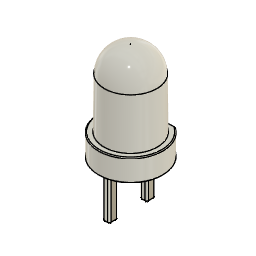
3mm (Autodesk Fusion 360 design; units mm, degrees)
Autodesk Fusion 360 part; units mm, degrees
sketch "Sketch1" plane through (0, 0, 0) normal (0, 0, 1) x (1, 0, 0)
  circle A0 centre (0, 0) radius 1.8
  line L0 (0, 0) -> (0, -1.8)
  line L1 (0, -1.8) -> (0, 1.5)
  line L2 (0, 1.5) -> (-0.995, 1.5)
  line L3 (0, 1.5) -> (0.995, 1.5)
  circle A1 centre (0, 0) radius 1.5
  dimension "d1" = 3.6
  dimension "d2" = 3.3
  dimension "d3" = 3
  constraint coincident A0.centre L0.start
  constraint coincident A0 L0.end
  constraint vertical L0
  constraint parallel L0 L1
  constraint coincident A0 L2.end
  constraint perpendicular L1 L2
  constraint coincident A0 L3.end
  constraint perpendicular L1 L3
  constraint concentric A0 A1
  measures "d1" diameter of A0
  measures "d2" distance of L0.end L1.end
  measures "d3" diameter of A1
extrude "Extrude1" add sketch "Sketch1" along normal blind 5.5 contours L0 L1 A1 | L0 L1 A1
extrude "Extrude2" add sketch "Sketch1" along normal blind 1.25 contours A0 L0 L1 L3 A1 | A0 L0 L1 L2 A1
chamfer "Chamfer1" distance 0.05 distance2 4.25 1 edges at (-1.3985, -0.5424, 5.5) measured on face at (0.4379, -0.6128, 5.5)
fillet "Fillet1" radius 0.05 5 edges at (0, -1.8, 1.25) (0.4975, 1.5, 1.25) (-0.4975, 1.5, 1.25) (0, -1.8, 0) (0, 1.5, 0)
fillet "Fillet2" radius 1.45 1 edges at (-1.3519, 0.5243, 5.5)
sketch "Sketch2" plane through (0, 0, 0) normal (0, 0, -1) x (1, 0, 0)
  line L0 (-0.9798, -1.45) -> (0.9798, -1.45)
  arc A0 (0.9798, -1.45) -> (-0.9798, -1.45) centre (0, 0) ccw
  line L1 (-0.2, -1.2) -> (0.2, -1.2)
  line L2 (0.2, -1.2) -> (0.2, -0.7)
  line L3 (0.2, -0.7) -> (-0.2, -0.7)
  line L4 (-0.2, -0.7) -> (-0.2, -1.2)
  line L5 (-0.2, -1.2) -> (0.2, -0.7) construction
  line L6 (0.2, -1.2) -> (-0.2, -0.7) construction
  line L7 (0, 0) -> (0, -1.45)
  line L8 (0, 0) -> (0, 1.75)
  line L9 (20, 0) -> (2.5, 0)
  arc A1 (0.9487, -1.35) -> (-0.9487, -1.35) centre (0, 0) ccw
  line L10 (-0.9487, -1.35) -> (0.9487, -1.35)
  line L11 (-0.2, 0.9) -> (0.2, 0.9)
  line L12 (0.2, 0.9) -> (0.2, 1.4)
  line L13 (0.2, 1.4) -> (-0.2, 1.4)
  line L14 (-0.2, 1.4) -> (-0.2, 0.9)
  line L15 (-0.2, 0.9) -> (0.2, 1.4) construction
  line L16 (0.2, 0.9) -> (-0.2, 1.4) construction
  point P0 (0, -0.95)
  point P1 (0, 1.15)
  dimension "d14" = 0.4
  dimension "d15" = 0.5
  dimension "d16" = 0.5
  dimension "d17" = -0.1
  dimension "d18" = 0.4
  dimension "d19" = 0.5
  dimension "d20" = 1.15
  constraint horizontal L1
  constraint perpendicular L1 L2
  constraint parallel L1 L3
  constraint parallel L2 L4
  constraint coincident L5 P0
  constraint coincident L6 P0
  constraint coincident A0.centre L7.start
  constraint midpoint L0 L7.end
  constraint midpoint A0 L8.end
  constraint coincident P0 L7
  constraint horizontal L11
  constraint perpendicular L11 L12
  constraint parallel L11 L13
  constraint parallel L12 L14
  constraint coincident L15 P1
  constraint coincident L16 P1
  constraint coincident L8 P1
  measures "d14" distance of L2.end L3.end
  measures "d15" distance of L1.end L2.end
  measures "d16" distance of L0 P0
  measures "d18" distance of L12.end L13.end
  measures "d19" distance of L11.end L12.end
  measures "d20" distance of A0.centre P1
extrude "Extrude3" cut sketch "Sketch2" against normal blind 0.3 contours L1 L3 L4 L7 L8 A1 L10 L11 L13 L14 | L1 L2 L3 L7 L8 A1 L10 L11 L12 L13
chamfer "Chamfer2" distance 0.05 distance2 0.3 1 edges at (0, -1.65, 0) measured on face at (0.3162, 1.4167, 0)
extrude "Extrude4" add 1 faces at (0.0667, 0.8667, 0) along direction (0, 0, -1) blind 2.5
extrude "Extrude5" add 1 faces at (-0.0667, -1.0667, 0) along direction (0, 0, -1) blind 2.5
fillet "Fillet3" radius 0.05 2 edges at (0, -1.7, 0) (0, 1.35, 0)
fillet "Fillet4" radius 0.1 8 edges at (0.2, 0.7, -1.1) (-0.2, 0.7, -1.1) (0.2, 1.2, -1.1) (0.2, -0.9, -1.1) (0.2, -1.4, -1.1) (-0.2, -1.4, -1.1) (-0.2, -0.9, -1.1) (-0.2, 1.2, -1.1) 2 faces at (-0.0667, -1.0667, -2.5) (0.0667, 0.8667, -2.5)
fillet "Fillet5" radius 0.2 16 edges at (0, 0.7, 0.3) (-0.1707, 0.7293, 0.3) (-0.2, 0.95, 0.3) (-0.1707, 1.1707, 0.3) (0, 1.2, 0.3) (0.1707, 1.1707, 0.3) (0.2, 0.95, 0.3) (0.1707, 0.7293, 0.3) (0, -1.4, 0.3) (-0.1707, -1.3707, 0.3) (-0.2, -1.15, 0.3) (-0.1707, -0.9293, 0.3) (0, -0.9, 0.3) (0.1707, -0.9293, 0.3) (0.2, -1.15, 0.3) (0.1707, -1.3707, 0.3)
named bodies: "White_3mm"
